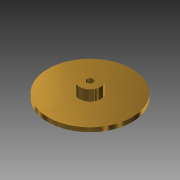
# Autodesk Inventor part: Gear4_S50B 80B+0203
Saved by Autodesk Inventor 2015 (Build 190159000, 159)
## iProperties
Created: 2013-10-31
Part Number: Gear4_S50B 80B+0203
Material: 真鍮
Document SubType Name: Modeling
Designer: kenta
Density: 8.49 g/cm^3
Appearance: 真鍮 - つや出し
Mass: 24.435 g
Surface Area: 29.908 cm^2
Volume: 2.87809 cm^3
Author: kenta
Autodesk Inventor part; units mm, degrees
ref_plane "YZ Plane" through (0, 0, 0) normal (1, 0, 0) x (0, 1, 0)
ref_plane "XZ Plane" through (0, 0, 0) normal (0, 1, 0) x (-1, 0, 0)
ref_plane "XY Plane" through (0, 0, 0) normal (0, 0, 1) x (1, 0, 0)
sketch "スケッチ4" plane through (0, 0, 0) normal (0, 0, 1) x (1, 0, 0)
  circle A0 centre (0, 0) radius 20
  dimension "d22" = 40
  constraints: 1 centre point, 1 coincident
  measures "d22" diameter of A0
extrude "押し出し3" add sketch "スケッチ4" along normal blind 2
sketch "スケッチ5" plane through (0, 0, 2) normal (0, 0, 1) x (1, 0, 0)
  circle A0 centre (0, 0) radius 5
  dimension "d25" = 10
  constraints: 1 centre point, 1 coincident
  measures "d25" diameter of A0
extrude "押し出し4" add sketch "スケッチ5" along normal blind 5
sketch "スケッチ6" plane through (0, 0, 0) normal (0, 0, -1) x (-1, 0, 0)
  circle A0 centre (0, 0) radius 4
  dimension "d28" = 8
  constraints: 1 centre point, 1 coincident
  measures "d28" diameter of A0
extrude "押し出し5" add sketch "スケッチ6" along normal blind 0.5
sketch "スケッチ7" plane through (0, 0, 7) normal (0, 0, 1) x (1, 0, 0)
  circle A0 centre (0, 0) radius 1.5
  dimension "d31" = 3
  constraints: 1 centre point, 1 coincident
  measures "d31" diameter of A0
extrude "押し出し6" cut sketch "スケッチ7" against normal blind 10
